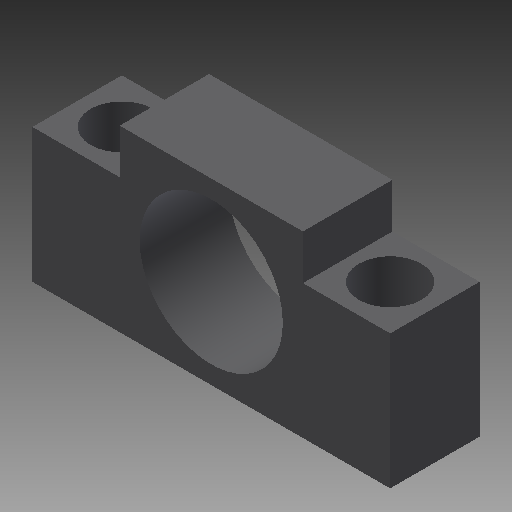
# Autodesk Inventor part: BF 15 Part1
Saved by Autodesk Inventor 2018 (Build 220112000, 112)
## iProperties
Category: PARTsolutions
Company: THK
Created: 2017-05-30
Part Number: BF 15 Part1
Catalog Web Link: www.cadenas.de
Description: Supported side type BF-Part1-
Vendor: THK
Document SubType Name: Modeling
Designer: psAdmin
Manufacturer: THK
Mass: 41.5867 g
Surface Area: 127.439 cm^2
Volume: 41.5867 cm^3
Density: 1 g/cm^3
Material: Generic
Appearance: PSOLRGB-192-192-192
PSOL_IDENT_0: {$CADENAS_DATA\23d-libs\thk\fed_screw\ball_screw\ball_screw_peripheral\suport_unit\supported_bf_1.pr
PSOL_IDENT_1: j},186 {VTYP=3D},{NB=BF 15 Part1},{LINA=BF 15 Part1},{NN=Supported side type BF-Part1},{DATE=16.05.2
PSOL_IDENT_2: 017 06:09:50},{GEOMDATE=08.02.2016 08:57:00},{VERSION=},{LINEID=30},{LINESUBID=-1},{WBVAR=}  {NB=BF
PSOL_IDENT_3: 15 Part1},{LINA=BF 15 Part1},{KT=DUMMY},{IDNR=},{MN=BF 15},{SD=15.000},{L=20.000},{B=70.000},{H=48.0
PSOL_IDENT_4: 00},{SB=35.000},{SH1=28.000},{B1=40.000},{H1=38.000},{E=18.000},{SD3=5.500},{P=54.000},{SD1=6.600},{
PSOL_IDENT_5: SD2=11.000},{SH=6.500},{DK=30.000},{L4=3.500},{SD4=20.000},{D=28.000},{DD=25.000},{P1=1.500},{B2=38.
PSOL_IDENT_6: 000},{D1=7.800},{DX=32.000}
NN: Supported side type BF-Part1
NB: BF 15 Part1
NBSYN: $MN. Part1
LINA: BF 15 Part1
MN: BF 15
SD: 15.000
L: 20.000
B: 70.000
H: 48.000
SB: 35.000
SH1: 28.000
B1: 40.000
H1: 38.000
E: 18.000
SD3: 5.500
P: 54.000
SD1: 6.600
SD2: 11.000
SH: 6.500
DK: 30.000
L4: 3.500
SD4: 20.000
D: 28.000
DD: 25.000
P1: 1.500
B2: 38.000
D1: 7.800
DX: 32.000
SUPPLIER: THK
ARTICLENO: BF 15 Part1
BOMINFO: BF 15 Part1
CREATOR: CADENAS GmbH
Title: BF 15 Part1
Author: Cadenas PARTsolutions
Autodesk Inventor part; units mm, degrees
ref_plane "YZ Plane" through (0, 0, 0) normal (1, 0, 0) x (0, 1, 0)
ref_plane "XZ Plane" through (0, 0, 0) normal (0, 1, 0) x (-1, 0, 0)
ref_plane "XY Plane" through (0, 0, 0) normal (0, 0, 1) x (1, 0, 0)
sketch "Sketch_1" plane through (0, 0, 0) normal (0, 0, 1) x (1, 0, 0)
  line L0 (-40.6072, -34.688) -> (39.3928, -34.688)
  line L1 (39.3928, -34.688) -> (39.3928, -4.688)
  line L2 (39.3928, -4.688) -> (19.8928, -4.688)
  line L3 (19.8928, -4.688) -> (19.8928, 5.312)
  line L4 (19.8928, 5.312) -> (-21.1072, 5.312)
  line L5 (-21.1072, 5.312) -> (-21.1072, -4.688)
  line L6 (-21.1072, -4.688) -> (-40.6072, -4.688)
  line L7 (-40.6072, -4.688) -> (-40.6072, -34.688)
  line L8 (-0.6072, -34.688) -> (-0.6072, 5.312) construction
  dimension "d24" = 80
  dimension "d25" = 40
  dimension "d26" = 10
  dimension "d27" = 10
  dimension "d28" = 41
  constraints: 18 end point, 3 vertical, 2 midpoint, 1 horizontal
  measures "d24" distance between parallel lines of L1 L7
  measures "d25" distance between parallel lines of L0 L4
  measures "d26" distance between parallel lines of L4 L6
  measures "d27" distance between parallel lines of L2 L4
  measures "d28" distance of L3.end L4.end
extrude "Extrusion1" add sketch "Sketch_1" against normal blind 20
sketch "Sketch2" plane through (19.8928, -4.688, 0) normal (0, 1, 0) x (1, 0, 0)
  line L0 (9.5, 10) -> (19.5, 10) construction
  line L1 (19.5, 0) -> (19.5, 20) projected
  dimension "d31" = 10
  constraints: 2 end point, 1 horizontal, 1 midpoint
  measures "d31" distance of L0.start L0.end
hole "Hole1" at (29.3928, -4.688, -10) direction (0, -1, 0) diameter 9 end through all counterbore diameter 14 counterbore depth 11
sketch "Sketch3" plane through (-40.6072, -4.688, 0) normal (0, 1, 0) x (1, 0, 0)
  line L0 (10, 10) -> (0, 10) construction
  line L1 (0, 0) -> (0, 20) projected
  dimension "d30" = 10
  constraints: 2 end point, 1 horizontal, 1 midpoint
  measures "d30" distance of L0.start L0.end
hole "Hole2" at (-30.6072, -4.688, -10) direction (0, -1, 0) diameter 9 end through all counterbore diameter 14 counterbore depth 11
sketch "Sketch4" plane through (0, 0, 0) normal (0, 0, 1) x (1, 0, 0)
  line L0 (-0.6072, -14.688) -> (-0.6072, 5.312) construction
  line L1 (19.8928, 5.312) -> (-21.1072, 5.312) projected
  dimension "d29" = 20
  constraints: 2 end point, 1 midpoint, 1 vertical
  measures "d29" distance of L0.start L0.end
hole "Hole3" at (-0.6072, -14.688, 0) direction (0, 0, -1) diameter 32 depth 20
ref_plane "bf_1_XY" through (0, 0, 0) normal (0, 0, 1) x (1, 0, 0)
ref_plane "bf_1_YZ" through (0, 0, 0) normal (1, 0, 0) x (0, 1, 0)
ref_plane "bf_1_ZX" through (0, 0, 0) normal (0, 1, 0) x (0, 0, 1)
ref_plane "bf_2x_XY" through (0, 0, -10) normal (0, 0, 1) x (1, 0, 0)
ref_plane "bf_2x_YZ" through (0, 0, -10) normal (1, 0, 0) x (0, 1, 0)
ref_plane "bf_2x_ZX" through (0, 0, -10) normal (0, 1, 0) x (0, 0, 1)
body "Solid1"
